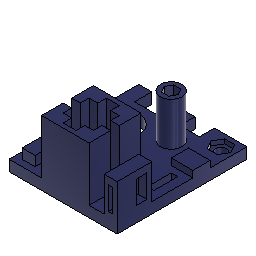
Valkayrie calibration part (Autodesk Fusion 360 design; units mm, degrees)
Autodesk Fusion 360 part; units mm, degrees
sketch "Sketch1" plane through (0, 0, 0) normal (0, 0, 1) x (1, 0, 0)
  circle A0 centre (-13, 10) radius 8.1
  line L0 (6.6454, 17.85) -> (3.3546, 17.85)
  line L1 (3.3546, 17.85) -> (1.7091, 15)
  line L2 (1.7091, 15) -> (3.3546, 12.15)
  line L3 (3.3546, 12.15) -> (6.6454, 12.15)
  line L4 (6.6454, 12.15) -> (8.2909, 15)
  line L5 (8.2909, 15) -> (6.6454, 17.85)
  circle A1 centre (-3, 25) radius 1.6
  line L6 (-25, -30) -> (-25, 30)
  line L7 (25, 30) -> (25, -30)
  line L8 (25, -30) -> (-25, 30) construction
  line L9 (23.6188, 24) -> (21.3094, 28)
  line L10 (21.3094, 28) -> (16.6906, 28)
  line L11 (16.6906, 28) -> (14.3812, 24)
  line L12 (14.3812, 24) -> (16.6906, 20)
  line L13 (16.6906, 20) -> (21.3094, 20)
  line L14 (21.3094, 20) -> (23.6188, 24)
  circle A2 centre (19, 24) radius 2.55
  line L15 (-22, -17) -> (-16, -17)
  line L16 (-16, -17) -> (-16, -27)
  line L17 (-16, -27) -> (-22, -27)
  line L18 (-22, -27) -> (-22, -17)
  circle A3 centre (0, 0) radius 2.5
  circle A4 centre (0, 0) radius 4
  line L19 (18, -9) -> (21, -9)
  line L20 (21, -9) -> (21, 2)
  line L21 (21, 2) -> (18, 2)
  line L22 (18, 2) -> (18, -9)
  line L23 (25, -30) -> (-25, -30)
  line L24 (1, 30) -> (1, 23)
  line L25 (1, 23) -> (10, 23)
  line L26 (10, 23) -> (10, 30)
  line L27 (10, 30) -> (25, 30)
  line L28 (-7, 30) -> (-7, 22)
  line L29 (-7, 22) -> (-19, 22)
  line L30 (-19, 22) -> (-19, 30)
  line L31 (25, 13) -> (15, 13)
  line L32 (15, 13) -> (15, 5)
  line L33 (15, 5) -> (25, 5)
  line L34 (25, 5) -> (25, 13)
  line L35 (-25, 30) -> (-19, 30)
  line L36 (-7, 30) -> (1, 30)
  line L37 (-25, -30) -> (-16, -19.2) construction
  circle A5 centre (5, 15) radius 5
  line L38 (-3, 30) -> (-3, 25) construction
  point P0 (5, 15)
  point P1 (19, 24)
  dimension "d1" = 16.2
  dimension "d2" = 2.85
  dimension "d3" = 3.2
  dimension "d4" = 50
  dimension "d5" = 60
  dimension "d11" = 4
  dimension "d12" = 5.1
  dimension "d18" = 6
  dimension "d19" = 10
  dimension "d23" = 5
  dimension "d24" = 8
  dimension "d29" = 3
  dimension "d30" = 11
  dimension "d36" = 9
  dimension "d37" = 7
  dimension "d68" = 8
  dimension "d69" = 8
  dimension "d70" = 3
  dimension "d71" = 3
  dimension "d72" = 35
  dimension "d73" = 8
  dimension "d74" = 10
  dimension "d76" = 20
  dimension "d77" = 12
  dimension "d78" = 12
  dimension "d79" = 6
  dimension "d80" = 10
  dimension "d81" = 6
  dimension "d82" = 6
  dimension "d83" = 25
  dimension "d84" = 15
  dimension "d85" = 20
  dimension "d86" = 4
  dimension "d88" = 28
  dimension "d89" = 5
  constraint horizontal L4.end P0
  constraint horizontal L23
  constraint perpendicular L6 L23
  constraint parallel L23 L35
  constraint parallel L6 L7
  constraint coincident L8 A3.centre
  constraint coincident A3.centre L37
  constraint horizontal L15
  constraint vertical L16
  constraint horizontal L17
  constraint vertical L18
  constraint concentric A3 A4
  constraint horizontal L19
  constraint vertical L20
  constraint horizontal L21
  constraint vertical L22
  constraint perpendicular L24 L35
  constraint perpendicular L24 L25
  constraint coincident L26.end L35
  constraint perpendicular L26 L35
  constraint collinear L27 L35
  constraint vertical L28
  constraint horizontal L29
  constraint vertical L30
  constraint horizontal L31
  constraint vertical L32
  constraint horizontal L33
  constraint vertical L34
  constraint coincident P1 A2.centre
  constraint horizontal L13
  constraint collinear L35 L36
  constraint coincident L16 L37.end
  constraint coincident P0 A5.centre
  constraint coincident A3.centre A4.centre
  constraint midpoint L36 L38.start
  constraint coincident A1.centre L38.end
  constraint vertical L38
  constraint collinear L7 L34
  measures "d1" diameter of A0
  measures "d2" distance of P0 L5
  measures "d3" diameter of A1
  measures "d4" distance of L6.end L7.start
  measures "d5" distance of L6.start L6.end
  measures "d11" distance of P1 L14
  measures "d12" diameter of A2
  measures "d18" distance of L15.start L15.end
  measures "d19" distance of L15.start L17.end
  measures "d23" diameter of A3
  measures "d24" diameter of A4
  measures "d29" distance of L19.start L19.end
  measures "d30" distance of L19.start L21.end
  measures "d36" distance of L24.end L25.end
  measures "d37" distance of L25.end L26.end
  measures "d68" distance of L30.end L29.end
  measures "d69" distance of L24 L28
  measures "d70" horizontal distance of L6.start L17.end
  measures "d71" vertical distance of L6.start L17.end
  measures "d72" vertical distance of L7.end L33.end
  measures "d73" distance of L31.start L33.end
  measures "d74" distance of L32.end L33.end
  measures "d76" vertical distance of A0.centre L6.end
  measures "d77" horizontal distance of A0.centre L6.end
  measures "d78" distance of L28 L30
  measures "d79" distance of L6 L30
  measures "d80" diameter of A5
  measures "d81" vertical distance of L7.start P1
  measures "d82" horizontal distance of L7.start P1
  measures "d83" distance of L7 A3.centre
  measures "d84" vertical distance of L7.start P0
  measures "d85" horizontal distance of L7.start P0
  measures "d86" horizontal distance of L7.start L20.end
  measures "d88" vertical distance of L7.start L20.end
  measures "d89" vertical distance of A1.centre L6.end
extrude "Extrude1" add sketch "Sketch1" along normal blind 5 contours L6 L7 L23 L24 L25 L26 L27 L28 L29 L30 L31 L32 L33 L35 L36 | L7 L31 L32 L33 L34 | L9 L10 L11 L12 L13 L14 | A2 | L15 L16 L17 L18 | A3 | A4 | L19 L20 L21 L22 | A5
extrude "Extrude2" add sketch "Sketch1" along normal blind 2.5 contours L0 L1 L2 L3 L4 L5
extrude "Extrude3" cut sketch "Sketch1" along normal blind 6.924 from surface at 3 contours L9 L10 L11 L12 L13 L14
extrude "Extrude4" cut sketch "Sketch1" along normal blind 10.975 contours A2
extrude "Extrude5" add sketch "Sketch1" along normal blind 4.5 from surface at 5 contours L15 L16 L17 L18
extrude "Extrude6" add sketch "Sketch1" along normal blind 17 contours A4
extrude "Extrude7" cut sketch "Sketch1" along normal blind 37.615 contours A3
extrude "Extrude8" cut sketch "Sketch1" along normal blind 27.204 contours L19 L20 L21 L22
chamfer "Chamfer1" distance 1 angle 45 4 edges at (18, -3.5, 0) (19.5, -9, 0) (21, -3.5, 0) (19.5, 2, 0)
sketch "Sketch2" plane through (0, 0, 5) normal (0, 0, 1) x (-1, 0, 0)
  line L0 (-18, -2) -> (-21, -2)
  line L1 (-21, -2) -> (-21, 9)
  line L2 (-21, 9) -> (-18, 9)
  line L3 (-18, 9) -> (-18, -2)
  line L4 (-21.3094, -20) -> (-16.6906, -20)
  line L5 (-16.6906, -20) -> (-14.3812, -24)
  line L6 (-14.3812, -24) -> (-16.6906, -28)
  line L7 (-16.6906, -28) -> (-21.3094, -28)
  line L8 (-21.3094, -28) -> (-23.6188, -24)
  line L9 (-23.6188, -24) -> (-21.3094, -20)
  line L10 (-6.6454, -17.85) -> (-8.2909, -15)
  line L11 (-8.2909, -15) -> (-6.6454, -12.15)
  line L12 (-6.6454, -12.15) -> (-3.3546, -12.15)
  line L13 (-3.3546, -12.15) -> (-1.7091, -15)
  line L14 (-1.7091, -15) -> (-3.3546, -17.85)
  line L15 (-3.3546, -17.85) -> (-6.6454, -17.85)
  circle A0 centre (3, -25) radius 1.6
  circle A1 centre (13, -10) radius 8.1
  line L16 (-25, 30) -> (-25, -30)
  line L17 (19, -30) -> (25, -30)
  line L18 (-10, -30) -> (-10, -23)
  line L19 (-10, -23) -> (-1, -23)
  line L20 (-1, -23) -> (-1, -30)
  line L21 (-1, -30) -> (7, -30)
  line L22 (25, -30) -> (25, 30)
  line L23 (25, 30) -> (-25, 30)
  line L24 (22, 27) -> (22, 17)
  line L25 (22, 17) -> (16, 17)
  line L26 (16, 17) -> (16, 27)
  line L27 (16, 27) -> (22, 27)
  circle A2 centre (0, 0) radius 4
  line L28 (-25, 30) -> (-19, 30)
  line L29 (-19, 30) -> (-19, 14)
  line L30 (-19, 14) -> (-25, 14)
  line L31 (-25, 14) -> (-25, 30)
  line L32 (7, -22) -> (19, -22)
  line L33 (19, -22) -> (19, -30)
  line L34 (7, -30) -> (7, -22)
  line L35 (-25, -30) -> (-10, -30)
  dimension "d38" = 6
  dimension "d39" = 16
  constraint horizontal L28
  constraint vertical L29
  constraint horizontal L30
  constraint vertical L31
  constraint coincident L16.start L23.end
  measures "d38" distance of L16.start L28.end
  measures "d39" distance of L28.end L29.end
extrude "Extrude9" add sketch "Sketch2" along normal blind 16 contours L16 L23 L28 L29 L30 L31
sketch "Sketch3" plane through (0, -30, 0) normal (0, -1, 0) x (1, 0, 0)
  line L0 (-25, 0) -> (25, 0)
  line L1 (25, 0) -> (25, 21)
  line L2 (25, 21) -> (19, 21)
  line L3 (19, 21) -> (19, 5)
  line L4 (19, 5) -> (-25, 5)
  line L5 (20.9088, 17.5998) -> (22.8502, 17.5998)
  line L6 (22.8502, 17.5998) -> (22.8502, 7.0605)
  line L7 (22.8502, 7.0605) -> (20.9088, 7.0605)
  line L8 (20.9088, 7.0605) -> (20.9088, 17.5998)
  line L9 (-25, 5) -> (-25, 0)
  constraint horizontal L5
  constraint vertical L6
  constraint horizontal L7
  constraint vertical L8
extrude "Extrude10" cut sketch "Sketch3" against normal blind 13.742 contours L5 L6 L7 L8
sketch "Sketch4" plane through (25, 0, 0) normal (1, 0, 0) x (0, 1, 0)
  line L0 (-30, 0) -> (30, 0)
  line L1 (30, 0) -> (30, 5)
  line L2 (30, 5) -> (-14, 5)
  line L3 (-14, 5) -> (-14, 21)
  line L4 (-14, 21) -> (-30, 21)
  line L5 (-30, 21) -> (-30, 0)
  line L6 (-16.258, 17.5998) -> (-21.1975, 17.5998)
  line L7 (-21.1975, 17.5998) -> (-21.1975, 7.0605)
  line L8 (-21.1975, 7.0605) -> (-16.258, 7.0605)
  line L9 (-16.258, 7.0605) -> (-16.258, 17.5998)
  line L10 (-30, 7.0605) -> (-16.258, 7.0605)
  point P0 (-16.258, 17.5998)
  constraint horizontal L6
  constraint vertical L7
  constraint horizontal L8
  constraint vertical L9
  constraint coincident L7.end L10
  constraint coincident P0 L6.start
extrude "Extrude11" cut sketch "Sketch4" against normal blind 4.091 contours L6 L7 L8 L9 L10
sketch "Sketch5" plane through (-25, 0, 0) normal (-1, 0, 0) x (0, -1, 0)
  line L0 (-30, 0) -> (30, 0)
  line L1 (30, 0) -> (30, 5)
  line L2 (30, 5) -> (-30, 5)
  line L3 (-30, 5) -> (-30, 0)
  line L4 (9, 1) -> (3.1, 1)
  line L5 (3.1, 1) -> (3.1, 4)
  line L6 (3.1, 4) -> (9, 4)
  line L7 (9, 4) -> (9, 1)
  line L8 (9, 1) -> (3.1, 4) construction
  line L9 (3.1, 1) -> (9, 4) construction
  line L10 (2.0114, 5) -> (2.0114, 0) construction
  point P0 (6.05, 2.5)
  point P1 (9, 1)
  dimension "d46" = 5.9
  dimension "d47" = 3
  constraint horizontal L4
  constraint perpendicular L4 L5
  constraint parallel L4 L6
  constraint parallel L5 L7
  constraint coincident P1 L4.start
  constraint coincident L8 P0
  constraint coincident L9 P0
  constraint coincident L2 L10.start
  constraint coincident L0 L10.end
  constraint perpendicular L0 L10
  measures "d46" distance of L5 P1
  measures "d47" distance of P1 L6.end
extrude "Extrude12" cut sketch "Sketch5" against normal blind 7 contours L4 L5 L6 L7
sketch "Sketch6" plane through (0, 0, 5) normal (0, 0, 1) x (-1, 0, 0)
  circle A0 centre (0, 0) radius 4
  line L0 (22, 27) -> (22, 17)
  line L1 (22, 17) -> (16, 17)
  line L2 (16, 17) -> (16, 27)
  line L3 (16, 27) -> (22, 27)
  line L4 (-19, 30) -> (-19, 14)
  line L5 (-19, 14) -> (-25, 14)
  line L6 (-25, 14) -> (-25, -30)
  line L7 (-25, -30) -> (-10, -30)
  line L8 (-10, -30) -> (-10, -23)
  line L9 (-10, -23) -> (-1, -23)
  line L10 (-1, -23) -> (-1, -30)
  line L11 (-1, -30) -> (7, -30)
  line L12 (25, -30) -> (25, 30)
  line L13 (25, 30) -> (-19, 30)
  circle A1 centre (13, -10) radius 8.1
  circle A2 centre (3, -25) radius 1.6
  line L14 (-6.6454, -17.85) -> (-8.2909, -15)
  line L15 (-8.2909, -15) -> (-6.6454, -12.15)
  line L16 (-6.6454, -12.15) -> (-3.3546, -12.15)
  line L17 (-3.3546, -12.15) -> (-1.7091, -15)
  line L18 (-1.7091, -15) -> (-3.3546, -17.85)
  line L19 (-3.3546, -17.85) -> (-6.6454, -17.85)
  line L20 (-21.3094, -20) -> (-16.6906, -20)
  line L21 (-16.6906, -20) -> (-14.3812, -24)
  line L22 (-14.3812, -24) -> (-16.6906, -28)
  line L23 (-16.6906, -28) -> (-21.3094, -28)
  line L24 (-21.3094, -28) -> (-23.6188, -24)
  line L25 (-23.6188, -24) -> (-21.3094, -20)
  line L26 (-18, -2) -> (-21, -2)
  line L27 (-21, -2) -> (-21, 9)
  line L28 (-21, 9) -> (-18, 9)
  line L29 (-18, 9) -> (-18, -2)
  circle A3 centre (21.5, 2.0114) radius 2.55
  line L30 (7, -30) -> (7, -22)
  line L31 (7, -22) -> (19, -22)
  line L32 (19, -22) -> (19, -30)
  line L33 (19, -30) -> (25, -30)
  dimension "d50" = 5.1
  measures "d50" diameter of A3
extrude "Extrude13" cut sketch "Sketch6" against normal blind 7.937 contours A3
extrude "Extrude14" add sketch "Sketch1" along normal blind 25 contours A5
sketch "Sketch7" plane through (0, 0, 5) normal (0, 0, 1) x (-1, 0, 0)
  circle A0 centre (21.5, 2.0114) radius 2.55
  circle A1 centre (0, 0) radius 4
  line L0 (22, 27) -> (22, 17)
  line L1 (22, 17) -> (16, 17)
  line L2 (16, 17) -> (16, 27)
  line L3 (16, 27) -> (22, 27)
  line L4 (-19, 30) -> (-19, 14)
  line L5 (-19, 14) -> (-25, 14)
  line L6 (-25, 14) -> (-25, -30)
  line L7 (-25, -30) -> (-10, -30)
  line L8 (-10, -30) -> (-10, -23)
  line L9 (-10, -23) -> (-1, -23)
  line L10 (-1, -23) -> (-1, -30)
  line L11 (-1, -30) -> (7, -30)
  line L12 (25, -30) -> (25, 30)
  line L13 (25, 30) -> (-19, 30)
  circle A2 centre (13, -10) radius 8.1
  circle A3 centre (3, -25) radius 1.6
  line L14 (-21.3094, -20) -> (-16.6906, -20)
  line L15 (-16.6906, -20) -> (-14.3812, -24)
  line L16 (-14.3812, -24) -> (-16.6906, -28)
  line L17 (-16.6906, -28) -> (-21.3094, -28)
  line L18 (-21.3094, -28) -> (-23.6188, -24)
  line L19 (-23.6188, -24) -> (-21.3094, -20)
  line L20 (-21, -2) -> (-21, 9)
  line L21 (-21, 9) -> (-18, 9)
  line L22 (-18, 9) -> (-18, -2)
  line L23 (6, 12) -> (6, 16)
  line L24 (6, 16) -> (10, 16)
  line L25 (10, 16) -> (10, 6)
  line L26 (10, 6) -> (-12, 6)
  line L27 (-12, 6) -> (-12, 16)
  line L28 (-12, 16) -> (-8, 16)
  line L29 (-8, 16) -> (-8, 12)
  line L30 (-8, 12) -> (-4, 12)
  line L31 (-4, 12) -> (-4, 8)
  line L32 (-4, 8) -> (2, 8)
  line L33 (2, 8) -> (2, 12)
  line L34 (2, 12) -> (6, 12)
  line L35 (8.4631, 18) -> (-4.0451, 18) construction
  line L36 (-12, 20) -> (-8, 20)
  line L37 (-8, 20) -> (-8, 24)
  line L38 (-8, 24) -> (-4, 24)
  line L39 (-4, 24) -> (-4, 28)
  line L40 (-4, 28) -> (2, 28)
  line L41 (2, 28) -> (2, 24)
  line L42 (2, 24) -> (6, 24)
  line L43 (6, 24) -> (6, 20)
  line L44 (6, 20) -> (10, 20)
  line L45 (10, 20) -> (10, 30)
  line L46 (-12, 30) -> (-12, 20)
  line L47 (10, 30) -> (-12, 30)
  line L48 (7, -30) -> (7, -22)
  line L49 (7, -22) -> (19, -22)
  line L50 (19, -22) -> (19, -30)
  line L51 (19, -30) -> (25, -30)
  circle A4 centre (-5, -15) radius 5
  line L52 (-18, -2) -> (-21, -2)
  dimension "d55" = 22
  dimension "d56" = 15
  dimension "d57" = 10
  dimension "d58" = 4
  dimension "d59" = 4
  dimension "d60" = 4
  dimension "d61" = 4
  dimension "d62" = 6
  dimension "d64" = 4
  dimension "d66" = 12
  constraint parallel L2 L23
  constraint perpendicular L2 L24
  constraint perpendicular L24 L25
  constraint perpendicular L2 L26
  constraint perpendicular L26 L27
  constraint perpendicular L27 L28
  constraint perpendicular L28 L29
  constraint perpendicular L27 L30
  constraint parallel L30 L32
  constraint perpendicular L32 L33
  constraint perpendicular L30 L31
  constraint horizontal L34
  constraint equal L31 L33
  constraint equal L30 L34
  constraint equal L25 L27
  constraint symmetric L23.start L35 L42.end
  constraint symmetric L23.end L35 L43.end
  constraint symmetric L24.end L35 L44.end
  constraint symmetric L25.end L35 L45.end
  constraint symmetric L26.end L35 L46.start
  constraint symmetric L27.end L35 L36.start
  constraint symmetric L28.end L35 L36.end
  constraint symmetric L29.end L35 L37.end
  constraint symmetric L30.end L35 L38.end
  constraint symmetric L31.end L35 L39.end
  constraint symmetric L32.end L35 L40.end
  constraint symmetric L33.end L35 L41.end
  constraint collinear L13 L47
  measures "d55" distance of L25.end L26.end
  measures "d56" distance of L12 L25.end
  measures "d57" distance of L26.end L27.end
  measures "d58" distance of L27.end L28.end
  measures "d59" distance of L29.end L30.end
  measures "d60" distance of L28.end L29.end
  measures "d61" distance of L30.end L31.end
  measures "d62" distance of L31.end L32.end
  measures "d64" distance of L23.end L24.end
  measures "d66" distance of L26 L35
extrude "Extrude15" add sketch "Sketch7" along normal blind 25 contours L13 L36 L37 L38 L39 L40 L41 L42 L43 L44 L45 L46 L47 | L23 L24 L25 L26 L27 L28 L29 L30 L31 L32 L33 L34
extrude "Extrude16" add sketch "Sketch1" along normal blind 8 contours L7 L31 L32 L33 L34
equation "d2 = ( 5.7 / 2 ) * 1 mm"
equation "d11 = ( 8 / 2 ) * 1 mm"
